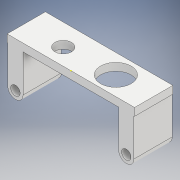
# Autodesk Inventor part: portaswitch
Saved by Autodesk Inventor 2018 (Build 220112000, 112)
## iProperties
Created: 2017-07-12
Part Number: portaswitch
Material: Default New Material(1)
Document SubType Name: Modeling
Designer: Vidal Villegas
Density: 1.13872 g/cm^3
Appearance: PLA
Mass: 5.11085 g
Surface Area: 34.3636 cm^2
Volume: 4.48824 cm^3
Author: Vidal Villegas
Autodesk Inventor part; units mm, degrees
ref_plane "YZ Plane" through (0, 0, 0) normal (1, 0, 0) x (0, 1, 0)
ref_plane "XZ Plane" through (0, 0, 0) normal (0, 1, 0) x (-1, 0, 0)
ref_plane "XY Plane" through (0, 0, 0) normal (0, 0, 1) x (1, 0, 0)
sketch "Sketch1" plane through (0, 0, 0) normal (0, 1, 0) x (-1, 0, 0)
  line L0 (25, 0) -> (-25, 0)
  line L1 (-25, 0) -> (-25, -3)
  line L2 (-25, -3) -> (25, -3)
  line L3 (25, -3) -> (25, 0)
  line L4 (0, 0) -> (0, -12.1399) construction
  line L5 (24.75, -3) -> (24.75, -17.6357)
  line L6 (18.75, -3) -> (18.75, -17.6357)
  arc A0 (18.75, -17.6357) -> (24.75, -17.6357) centre (21.75, -17.6357) ccw
  circle A1 centre (21.75, -17.6357) radius 1.85
  line L7 (-24.75, -3) -> (-24.75, -17.6357)
  line L8 (-18.75, -3) -> (-18.75, -17.6357)
  arc A2 (-24.75, -17.6357) -> (-18.75, -17.6357) centre (-21.75, -17.6357) ccw
  circle A3 centre (-21.75, -17.6357) radius 1.85
  line L9 (-24.75, -3) -> (-18.75, -3)
  dimension "d0" = 3
  dimension "d1" = 50
  dimension "d2" = 43.5
  dimension "d3" = 14.6357
  dimension "d4" = 3.7
  dimension "d5" = 3
  constraints: 20 end point, 6 symmetric about line, 4 centre point, 4 point on circle, 3 vertical, 2 coincident, 2 horizontal, 2 parallel, 2 point on line, 2 tangent, 1 horizontal alignment, 1 perpendicular, 3 other
  measures "d0" distance of L0.end L1.end
  measures "d1" distance of L0.start L0.end
  measures "d2" distance of A2.centre A0.centre
  measures "d3" distance from line of A0.centre L2
  measures "d4" diameter of A1
  measures "d5" radius of A0
extrude "Extrusion1" add sketch "Sketch1" along normal blind 15
sketch "Sketch2" plane through (-25, 0, 0) normal (0, 0, 1) x (1, 0, 0)
  line L0 (0, 0) -> (50, 0) projected
  line L1 (50, 0) -> (50, 15) projected
  line L2 (0, 15) -> (50, 15) projected
  line L3 (0, 0) -> (0, 15) projected
  circle A0 centre (15.5, 6.5) radius 3.25
  circle A1 centre (35.25, 7.4) radius 6
  line L4 (43.75, 0) -> (43.75, 15) projected
  point P0 (25, 0)
  point P1 (25, 0)
  point P2 (50, 7.5)
  point P3 (0, 7.5)
  dimension "d8" = 6.5
  dimension "d14" = 34.5
  dimension "d15" = 8.5
  dimension "d16" = 12
  dimension "d17" = 8.5
  dimension "d21" = 15
  dimension "d22" = 7.4
  constraints: 3 midpoint, 2 centre point
  measures "d8" diameter of A0
  measures "d14" distance from line of A0.centre L1
  measures "d15" distance from line of A0.centre L2
  measures "d16" diameter of A1
  measures "d17" distance from line of L4 A1.centre
  measures "d21" distance between parallel lines of L2 L0
  measures "d22" distance from line of A1.centre L0
extrude "Extrusion2" cut sketch "Sketch2" against normal through all contours A0
sketch "Sketch3" plane through (0, 0, 0) normal (0, -1, 0) x (1, 0, 0)
  point P0 (0, 0)
extrude "Extrusion3" cut sketch "Sketch2" against normal through all contours A1
body "Solid1"
